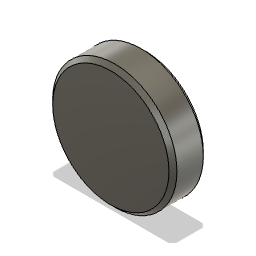
Magnet_Bump (Autodesk Fusion 360 design; units mm, degrees)
Autodesk Fusion 360 part; units mm, degrees
sketch "Sketch1" plane through (0, 0, 0) normal (0, 0, 1) x (1, 0, 0)
  circle A0 centre (0, 0) radius 7.775
  circle A1 centre (0, 0) radius 4.775
  dimension "d1" = 9.55
  dimension "d2" = 15.55
  constraint coincident A0.centre A1.centre
  constraint concentric A0 A1
  measures "d1" diameter of A1
  measures "d2" diameter of A0
extrude "Extrude1" add sketch "Sketch1" along normal blind 1 contours A0 | A1
extrude "Extrude2" add sketch "Sketch1" against normal blind 3.3
chamfer "Chamfer1" distance 0.5 angle 45 3 edges at (-7.2488, -2.8116, 1) (-7.2488, 2.8116, -3.3) (-4.4519, -1.7267, -3.3)
equation "d2 = d1 + 6 mm"
named bodies: "magnet_bump"
